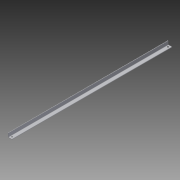
# Autodesk Inventor part: .05 in Aluminum Angle
Saved by Autodesk Inventor 2014 (Build 180170000, 170)
## iProperties
Created: 2014-01-05
Part Number: .05 in Aluminum Angle
Material: Aluminum 6061
Document SubType Name: Modeling
Designer: Michael
Density: 2.71 g/cm^3
Appearance: Aluminum - Flat
Author: Michael
Autodesk Inventor part; units mm, degrees
ref_plane "YZ Plane" through (0, 0, 0) normal (1, 0, 0) x (0, 1, 0)
ref_plane "XZ Plane" through (0, 0, 0) normal (0, 1, 0) x (-1, 0, 0)
ref_plane "XY Plane" through (0, 0, 0) normal (0, 0, 1) x (1, 0, 0)
sketch "Sketch1" plane through (0, 0, 0) normal (0, 0, 1) x (1, 0, 0)
  line L0 (0, 0) -> (12.7, 0)
  line L1 (12.7, 0) -> (12.7, 1.27)
  line L2 (12.7, 1.27) -> (1.27, 1.27)
  line L3 (1.27, 1.27) -> (1.27, 12.7)
  line L4 (1.27, 12.7) -> (0, 12.7)
  line L5 (0, 12.7) -> (0, 0)
  dimension "d0" = 12.7
  dimension "d1" = 1.27
  dimension "d2" = 11.43
  constraints: 12 end point, 4 perpendicular, 2 parallel, 1 horizontal
  measures "d0" distance of L0.start L0.end
  measures "d1" distance of L0.end L1.end
  measures "d2" distance of L1.end L2.end
extrude "Extrusion1" add sketch "Sketch1" along normal blind 508
fillet "Fillet1" radius 1.27 4 edges at (12.7, 1.27, 254) (1.27, 12.7, 254) (1.27, 1.27, 254) (0, 0, 254)
sketch "Sketch2" plane through (2.54, 1.27, 508) normal (0, 1, 0) x (1, 0, 0)
  line L0 (0, 0) -> (0, 508) projected
  line L1 (8.89, 0) -> (0, 0) projected
  line L2 (8.89, 508) -> (8.89, 0) projected
  circle A0 centre (3.81, 6.35) radius 2.4892
  line L3 (-2.54, 0) -> (-2.54, 508) projected
  line L4 (-2.54, 508) -> (-2.54, 0) projected
  line L5 (8.89, 254) -> (0, 254) construction
  circle A1 centre (3.81, 501.65) radius 2.4892
  dimension "d6" = 4.9784
  dimension "d7" = 6.35
  dimension "d8" = 6.35
  constraints: 2 centre point, 2 end point, 2 midpoint, 1 symmetric about line, 1 other
  measures "d6" diameter of A0
  measures "d7" distance from line of A0.centre L4
  measures "d8" distance from line of L1 A0.centre
extrude "Extrusion2" cut sketch "Sketch2" against normal blind 25.4
body "Solid1"
